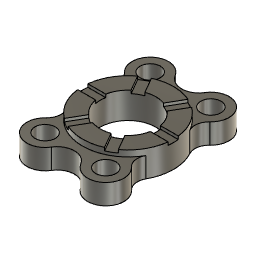
САПиП.АДМ2105.АбдулзагировМурад.Деталь1ЛР2 (Autodesk Fusion 360 design; units mm, degrees)
Autodesk Fusion 360 part; units mm, degrees
sketch "Sketch1" plane through (0, 0, 0) normal (0, 0, 1) x (1, 0, 0)
  circle A0 centre (0, 0) radius 27.5
  circle A1 centre (30, -51.9615) radius 10
  line L0 (0, 0) -> (0, -67.6601)
  line L1 (0, 0) -> (30, -51.9615) construction
  line L2 (0, 0) -> (10.1597, -17.5971) construction
  line L3 (0, 0) -> (20.3193, 0) construction
  arc A2 (39.4278, -21.6899) -> (42.203, -38.7295) centre (51.6942, -28.4379) ccw
  arc A3 (14.5714, -61.2329) -> (42.203, -38.7295) centre (30, -51.9615) ccw
  circle A4 centre (-30, -51.9615) radius 10
  arc A5 (-42.203, -38.7295) -> (-39.4278, -21.6899) centre (-51.6942, -28.4379) ccw
  arc A6 (14.5714, -61.2329) -> (-14.5714, -61.2329) centre (0, -69.9893) ccw
  arc A7 (-42.203, -38.7295) -> (-14.5714, -61.2329) centre (-30, -51.9615) ccw
  arc A8 (-14.5714, 61.2329) -> (-42.203, 38.7295) centre (-30, 51.9615) ccw
  arc A9 (-39.4278, 21.6899) -> (-42.203, 38.7295) centre (-51.6942, 28.4379) ccw
  circle A10 centre (-30, 51.9615) radius 10
  arc A11 (-14.5714, 61.2329) -> (14.5714, 61.2329) centre (0, 69.9893) ccw
  arc A12 (42.203, 38.7295) -> (14.5714, 61.2329) centre (30, 51.9615) ccw
  circle A13 centre (30, 51.9615) radius 10
  arc A14 (42.203, 38.7295) -> (39.4278, 21.6899) centre (51.6942, 28.4379) ccw
  arc A15 (39.4278, -21.6899) -> (39.4278, 21.6899) centre (0, 0) ccw
  arc A16 (-39.4278, 21.6899) -> (-39.4278, -21.6899) centre (0, 0) ccw
  dimension "d1" = 55
  dimension "d2" = 90
  dimension "d4" = 20
  dimension "d5" = 36
  dimension "d6" = 28
  dimension "d7" = 60
  dimension "d8" = 34
  constraint coincident A0.centre L0.start
  constraint vertical L0
  constraint coincident A1.centre L1.end
  constraint concentric A1 A3
  constraint tangent A2 A3
  constraint horizontal L3
  constraint parallel L1 L2
  constraint tangent A2 A15
  constraint symmetric A1 L0 A4
  constraint symmetric L0 A2.end A5.start
  constraint symmetric L0 A2.start A5.end
  constraint symmetric L0 A2 A5
  constraint symmetric L0 A3 A7
  constraint tangent A3 A6
  constraint tangent A6 A7
  constraint symmetric A1 L3 A13
  constraint symmetric L3 A2.end A12.start
  constraint symmetric L3 A2.start A14.end
  constraint symmetric L3 A2 A14
  constraint symmetric L3 A3 A12
  constraint symmetric L3 A5.start A8.end
  constraint symmetric L3 A4 A10
  constraint symmetric L3 A5.end A9.start
  constraint symmetric L3 A5 A9
  constraint symmetric L3 A6.end A8.start
  constraint symmetric L3 A3.start A11.end
  constraint symmetric L3 A6 A11
  constraint symmetric L3 A7 A8
  constraint concentric A15 A16
  measures "d1" diameter of A0
  measures "d2" diameter of A15
  measures "d4" diameter of A1
  measures "d5" diameter of A3
  measures "d6" diameter of A2
  measures "d7" angle of L2 L3
  measures "d8" diameter of A6
extrude "Extrude1" add sketch "Sketch1" along normal blind 20
sketch "Sketch2" plane through (0, 0, 20) normal (0, 0, 1) x (-1, 0, 0)
  circle A0 centre (30, 51.9615) radius 10
  circle A1 centre (30, -51.9615) radius 10
  circle A2 centre (-30, -51.9615) radius 10
  circle A3 centre (-30, 51.9615) radius 10
  circle A4 centre (0, 0) radius 27.5
  arc A5 (14.5714, -61.2329) -> (42.203, -38.7295) centre (30, -51.9615) ccw
  arc A6 (39.4278, -21.6899) -> (42.203, -38.7295) centre (51.6942, -28.4379) ccw
  arc A7 (39.4278, -21.6899) -> (39.4278, 21.6899) centre (0, 0) ccw
  arc A8 (42.203, 38.7295) -> (39.4278, 21.6899) centre (51.6942, 28.4379) ccw
  arc A9 (42.203, 38.7295) -> (14.5714, 61.2329) centre (30, 51.9615) ccw
  arc A10 (-14.5714, 61.2329) -> (14.5714, 61.2329) centre (0, 69.9893) ccw
  arc A11 (-14.5714, 61.2329) -> (-42.203, 38.7295) centre (-30, 51.9615) ccw
  arc A12 (-39.4278, 21.6899) -> (-42.203, 38.7295) centre (-51.6942, 28.4379) ccw
  arc A13 (-39.4278, 21.6899) -> (-39.4278, -21.6899) centre (0, 0) ccw
  arc A14 (-42.203, -38.7295) -> (-39.4278, -21.6899) centre (-51.6942, -28.4379) ccw
  arc A15 (-42.203, -38.7295) -> (-14.5714, -61.2329) centre (-30, -51.9615) ccw
  arc A16 (14.5714, -61.2329) -> (-14.5714, -61.2329) centre (0, -69.9893) ccw
  circle A17 centre (0, 0) radius 27.5
  circle A18 centre (0, 0) radius 45
  constraint coincident A4.centre A7.centre
  constraint concentric A4 A18
extrude "Extrude2" add sketch "Sketch2" along normal blind 3 contours A7 A13 A18
sketch "Sketch3" plane through (0, 0, 23) normal (0, 0, 1) x (-1, 0, 0)
  circle A0 centre (0, 0) radius 27.5
  circle A1 centre (0, 0) radius 45
  line L0 (0, 0) -> (45, 0) construction
  line L1 (45, 0) -> (45, -1)
  line L2 (44.7214, -5) -> (27.0416, -5)
  line L3 (44.7214, 5) -> (27.0416, 5)
  line L4 (26.6908, 36.2298) -> (17.8509, 20.9187)
  line L5 (18.0306, 41.2298) -> (9.1907, 25.9187)
  line L6 (-18.0306, 41.2298) -> (-9.1907, 25.9187)
  line L7 (-26.6908, 36.2298) -> (-17.8509, 20.9187)
  line L8 (-44.7214, 5) -> (-27.0416, 5)
  line L9 (-44.7214, -5) -> (-27.0416, -5)
  line L10 (-26.6908, -36.2298) -> (-17.8509, -20.9187)
  line L11 (-18.0306, -41.2298) -> (-9.1907, -25.9187)
  line L12 (18.0306, -41.2298) -> (9.1907, -25.9187)
  line L13 (26.6908, -36.2298) -> (17.8509, -20.9187)
  arc A2 (-9.1907, -25.9187) -> (9.1907, -25.9187) centre (0, 0) ccw
  arc A3 (-18.0306, -41.2298) -> (18.0306, -41.2298) centre (0, 0) ccw
  arc A4 (-44.7214, -5) -> (-26.6908, -36.2298) centre (0, 0) ccw
  arc A5 (-27.0416, -5) -> (-17.8509, -20.9187) centre (0, 0) ccw
  arc A6 (17.8509, -20.9187) -> (27.0416, -5) centre (0, 0) ccw
  arc A7 (26.6908, -36.2298) -> (44.7214, -5) centre (0, 0) ccw
  arc A8 (27.0416, 5) -> (17.8509, 20.9187) centre (0, 0) ccw
  arc A9 (9.1907, 25.9187) -> (-9.1907, 25.9187) centre (0, 0) ccw
  arc A10 (-17.8509, 20.9187) -> (-27.0416, 5) centre (0, 0) ccw
  arc A11 (-26.6908, 36.2298) -> (-44.7214, 5) centre (0, 0) ccw
  arc A12 (44.7214, 5) -> (26.6908, 36.2298) centre (0, 0) ccw
  arc A13 (18.0306, 41.2298) -> (-18.0306, 41.2298) centre (0, 0) ccw
  dimension "d15" = 360
  constraint coincident A0.centre A1.centre
  constraint coincident A1 L0.end
  constraint horizontal L0
  constraint tangent A1 L1
  constraint coincident A0 L2.end
  constraint coincident A1 L2.start
  constraint symmetric L0 L2.end L3.end
  constraint symmetric L0 L2.start L3.start
  constraint coincident L0.end A7
  constraint concentric A2 A6
  constraint concentric A3 A7
  constraint concentric A4 A7
  constraint concentric A5 A6
  constraint concentric A6 A8
  constraint concentric A7 A12
  constraint concentric A8 A9
  constraint concentric A9 A10
  constraint concentric A11 A12
  constraint concentric A12 A13
extrude "Extrude3" add sketch "Sketch3" along normal blind 3 contours A0 A1 L3 L4 A8 A12 | A0 A1 L2 L13 A6 A7 | A0 A1 L5 L6 A9 A13 | A0 A1 L11 L12 A2 A3 | A0 A1 L7 L8 A10 A11 | A0 A1 L9 L10 A4 A5
